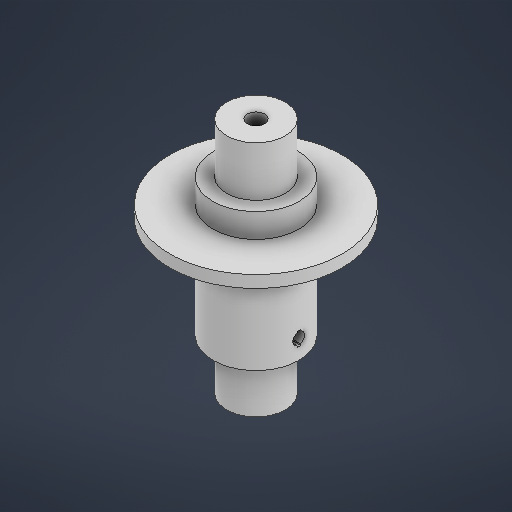
# Autodesk Inventor part: shaft for print
Saved by Autodesk Inventor 2025.2 (Build 292293000, 293)
## iProperties
Created: 2025-04-19
Part Number: shaft for print
Material: Generic
Document SubType Name: Modeling
Designer: klawy
Density: 1 g/cm^3
Appearance: Default
Author: klawy
Autodesk Inventor part; units mm, degrees
sketch "Sketch1" plane through (0, 0, 0) normal (0, 0, 1) x (1, 0, 0)
  line L0 (0, -16) -> (8.5, -16)
  line L1 (8.5, -16) -> (8.5, 16)
  line L2 (8.5, 16) -> (0, 16)
  line L3 (0, 16) -> (0, -16)
  line L4 (8.5, 4) -> (25, 4)
  line L5 (25, 4) -> (25, 1.5)
  line L6 (25, 1.5) -> (8.5, 1.5)
  line L7 (8.5, 1.5) -> (8.5, 4)
  line L8 (25, 1.5) -> (22, 1.5)
  line L9 (22, 1.5) -> (22, 0.5)
  line L10 (22, 0.5) -> (25, 0.5)
  line L11 (25, 0.5) -> (25, 1.5)
  line L12 (0, -22.4) -> (0, 22.4) construction
  line L13 (8.5, -16) -> (12.5, -16)
  line L14 (12.5, -16) -> (12.5, 1.5)
  line L15 (12.5, 1.5) -> (8.5, 1.5)
  line L16 (8.5, 1.5) -> (8.5, -16)
  point P0 (0, 0)
  point P1 (0, 0)
  point P2 (8.5, 1.5)
  point P3 (22, 1.5)
  dimension "d0" = 32
  dimension "d1" = 8.5
  dimension "d3" = 2.5
  dimension "d4" = 12
  dimension "d5" = 3
  dimension "d6" = 1
  dimension "d32" = 4
  dimension "d62" = 25
  constraints: 32 end point, 8 parallel, 4 horizontal, 4 perpendicular, 2 coincident, 2 point on line, 1 midpoint
  measures "d0" distance of L0.end L1.end
  measures "d1" distance of L1.end L2.end
  measures "d3" distance between parallel lines of L4 L6
  measures "d4" distance between parallel lines of L2 L4
  measures "d5" distance between parallel lines of L11 L9
  measures "d6" distance from line of L5.end L10
  measures "d32" distance between parallel lines of L1 L14
  measures "d62" distance between parallel lines of L12 L5
revolve "Revolution1" add sketch "Sketch1" angle 360 about axis through (0, -10, 0) along (0, 1, 0)
sketch "Sketch3" plane through (0, -16, 0) normal (0, -1, 0) x (1, 0, 0)
  circle A0 centre (0, 0) radius 2.621
  circle A1 centre (0, 0) radius 12.5 projected
  circle A2 centre (0, 0) radius 8.5 projected
  constraints: 1 centre point, 1 coincident
extrude "Extrusion1" add sketch "Sketch3" along normal blind 13 contours A0 | A1 | A2
sketch "Sketch4" plane through (0, -29, 0) normal (0, -1, 0) x (1, 0, 0)
  circle A0 centre (0, 0) radius 8.5
  circle A1 centre (0, 0) radius 12.5 projected
  dimension "d24" = 17
  constraints: 1 centre point, 1 coincident
  measures "d24" diameter of A0
extrude "Extrusion2" add sketch "Sketch4" along normal blind 15 contours A0
sketch "Sketch5" plane through (0, 16, 0) normal (0, 1, 0) x (1, 0, 0)
  circle A0 centre (0, 0) radius 8.5
  circle A1 centre (0, 0) radius 8.5 projected
  constraints: 2 coincident, 1 centre point, 1 concentric
extrude "Extrusion3" add sketch "Sketch5" along normal blind 10
sketch "Sketch6" plane through (0, 4, 0) normal (0, 1, 0) x (1, 0, 0)
  circle A0 centre (0, 0) radius 2.621 projected
  circle A1 centre (0, 0) radius 12.5
  circle A2 centre (0, 0) radius 8.5 projected
  dimension "d29" = 25
  constraints: 1 centre point, 1 coincident
  measures "d29" diameter of A1
extrude "Extrusion4" add sketch "Sketch6" along normal blind 7 contours A1
sketch "Sketch7" plane through (0, 26, 0) normal (0, 1, 0) x (1, 0, 0)
  point P0 (0, 0)
  point P1 (0, 0)
  constraints: 1 coincident
hole "Hole2" at (0, 26, 0) direction (0, -1, 0) diameter 3.4 end through all clearance for "Socket Head Cap Screw ISO 4762" size "M3" standard "ISO"
sketch "Sketch8" plane through (0, 26, 0) normal (0, 1, 0) x (1, 0, 0)
  circle A0 centre (0, 0) radius 2.5
  dimension "d41" = 5
  constraints: 1 centre point, 1 coincident
  measures "d41" diameter of A0
extrude "Extrusion5" cut sketch "Sketch8" against normal blind 7.5
sketch "Sketch9" plane through (0, -44, 0) normal (0, -1, 0) x (1, 0, 0)
  circle A0 centre (0, 0) radius 2.5
  dimension "d44" = 5
  constraints: 1 centre point, 1 coincident
  measures "d44" diameter of A0
extrude "Extrusion6" cut sketch "Sketch9" against normal blind 47.5
ref_plane "Work Plane1" through (12.5, 0, 0) normal (1, 0, 0) x (0, 1, 0)
sketch "Sketch10" plane through (12.5, 0, 0) normal (1, 0, 0) x (0, 1, 0)
  line L0 (26, -8.5) -> (26, 8.5) projected
  line L1 (-33.4, 0) -> (35.9, 0) projected
  point P0 (0, 0)
  point P1 (-23.5, 0)
  dimension "d54" = 49.5
  constraints: 1 point on line
  measures "d54" distance from line of point (-23.5, 0) L0
hole "Hole3" at (12.5, -23.5, 0) direction (-1, 0, 0) diameter 3.4 depth 8.8 tip angle 118 clearance for "Socket Head Cap Screw ISO 4762" size "M3" standard "ISO"
ref_plane "Work Plane2" through (7.5, 0, 0) normal (1, 0, 0) x (0, 1, 0)
sketch "Sketch13" plane through (7.5, 0, 0) normal (1, 0, 0) x (0, 1, 0)
  circle A0 centre (-23.5, 0) radius 1.7 projected
  circle A1 centre (-23.5, 0) radius 2.75 construction
  line L0 (-26.25, -1.5877) -> (-26.25, 1.5877)
  line L1 (-26.25, 1.5877) -> (-23.5, 3.1754)
  line L2 (-23.5, 3.1754) -> (-20.75, 1.5877) construction
  line L3 (-20.75, 1.5877) -> (-20.75, -1.5877) construction
  line L4 (-20.75, -1.5877) -> (-23.5, -3.1754) construction
  line L5 (-23.5, -3.1754) -> (-26.25, -1.5877)
  line L6 (-23.5, 3.1754) -> (-20.67, 3.1754)
  line L7 (-20.67, 3.1754) -> (-20.67, -3.1754)
  line L8 (-20.67, -3.1754) -> (-23.5, -3.1754)
  point P0 (0, 0)
  point P1 (-24.875, -2.3816)
  dimension "d64" = 5.5
  dimension "d92" = 0.08
  constraints: 18 end point, 2 coincident, 2 perpendicular, 1 midpoint, 1 vertical, 16 other
  measures "d92" distance between parallel lines of L3 L7
extrude "Extrusion7" cut sketch "Sketch13" against normal blind 2.48
ref_plane "Work Plane3" through (0, -36.5, 0) normal (0, -1, 0) x (1, 0, 0)
sketch "Sketch14" plane through (0, -36.5, 0) normal (0, -1, 0) x (1, 0, 0)
  circle A0 centre (0, 0) radius 2.5 projected
  circle A1 centre (0, 0) radius 8.5 projected
  constraints: 1 coincident
extrude "Extrusion8" add sketch "Sketch14" against normal blind 15 contours A0
sketch "Sketch15" plane through (0, -36.5, 0) normal (0, -1, 0) x (1, 0, 0)
  circle A0 centre (0, 0) radius 2.5 projected
  constraints: 1 coincident
hole "Hole4" at (0, -36.5, 0) direction (0, 1, 0) diameter 3.4 end through all clearance for "Countersunk Flat Head Screw ISO 2009/7046" size "M3" standard "ISO"
chamfer "Chamfer5" distance 0.8 angle 45 2 edges at (0, -21.5, 1.7) (0, -36.5, 1.7)
ref_plane "Work Plane4" through (0, -9, 0) normal (0, 1, 0) x (1, 0, 0)
ref_plane "Work Plane5" through (0, 13.5, 0) normal (0, 1, 0) x (1, 0, 0)
sketch "Sketch16" plane through (0, 13.5, 0) normal (0, 1, 0) x (1, 0, 0)
  circle A0 centre (0, 0) radius 2.75 construction
  line L0 (1.5877, 2.75) -> (3.1754, 0)
  line L1 (3.1754, 0) -> (1.5877, -2.75)
  line L2 (1.5877, -2.75) -> (-1.5877, -2.75)
  line L3 (-1.5877, -2.75) -> (-3.1754, 0)
  line L4 (-3.1754, 0) -> (-1.5877, 2.75)
  line L5 (-1.5877, 2.75) -> (1.5877, 2.75)
  point P0 (0, 2.75)
  dimension "d83" = 5.5
  constraints: 12 end point, 2 coincident, 1 horizontal, 1 midpoint, 1 vertical alignment, 15 other
extrude "Extrusion9" cut sketch "Sketch16" against normal blind 4.96
mirror "Mirror1" about plane through (0, -9, 0) normal (0, 1, 0) of "Extrusion9"
sketch "Sketch17" plane through (0, 26, 0) normal (0, 1, 0) x (1, 0, 0)
  circle A0 centre (0, 0) radius 2.5 projected
  circle A1 centre (0, 0) radius 8.5 projected
extrude "Extrusion10" cut sketch "Sketch17" against normal blind 0.5
sketch "Sketch18" plane through (0, -44, 0) normal (0, -1, 0) x (1, 0, 0)
  circle A0 centre (0, 0) radius 2.5 projected
  circle A1 centre (0, 0) radius 8.5 projected
extrude "Extrusion11" cut sketch "Sketch18" against normal blind 0.5
chamfer "Chamfer6" distance 0.8 angle 45 2 edges at (0, 18.5, -1.7) (0, 3.5, -1.7)
sketch "Sketch19" plane through (12.5, 0, 0) normal (1, 0, 0) x (0, 1, 0)
  circle A0 centre (-23.5, 0) radius 1.7 projected
  line L0 (-21.5, -0.5) -> (-25.5, -0.5)
  line L1 (-25.5, -0.5) -> (-25.5, 0.5)
  line L2 (-25.5, 0.5) -> (-21.5, 0.5)
  line L3 (-21.5, 0.5) -> (-21.5, -0.5)
  line L4 (-21.5, -0.5) -> (-25.5, 0.5) construction
  line L5 (-25.5, -0.5) -> (-21.5, 0.5) construction
  point P0 (0, 0)
  dimension "d96" = 4
  dimension "d97" = 1
  constraints: 12 end point, 2 midpoint, 2 parallel, 1 horizontal, 1 perpendicular
  measures "d96" distance of L1.end L2.end
  measures "d97" distance of L0.end L1.end
extrude "Extrusion12" cut sketch "Sketch19" against normal blind 8.5 contours A0 L0 L2 | A0 L2 L3 L0 | A0 L0 L1 L2
body "Solid1"
